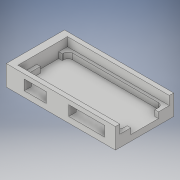
# Autodesk Inventor part: PiHolder
Saved by Autodesk Inventor 2019 (Build 230136000, 136)
## iProperties
Created: 2019-04-12
Part Number: PiHolder
Material: Generic
Document SubType Name: Modeling
Designer: Epsilon
Density: 1 g/cm^3
Appearance: Default
Author: Epsilon
Autodesk Inventor part; units mm, degrees
ref_plane "YZ Plane" through (0, 0, 0) normal (1, 0, 0) x (0, 1, 0)
ref_plane "XZ Plane" through (0, 0, 0) normal (0, 1, 0) x (-1, 0, 0)
ref_plane "XY Plane" through (0, 0, 0) normal (0, 0, 1) x (1, 0, 0)
sketch "Sketch2" plane through (0, 0, 0) normal (0, 1, 0) x (-1, 0, 0)
  line L0 (0, 0) -> (75, 0)
  line L1 (75, 0) -> (75, -40)
  line L2 (75, -40) -> (0, -40)
  line L3 (0, -40) -> (0, 0)
  dimension "d4" = 75
  dimension "d5" = 40
  constraints: 8 end point, 2 parallel, 1 horizontal, 1 perpendicular
  measures "d4" distance of L1.end L2.end
  measures "d5" distance of L0.end L1.end
extrude "Extrusion2" add sketch "Sketch2" along normal blind 14
sketch "Sketch4" plane through (0, 14, 0) normal (0, 1, 0) x (1, 0, 0)
  line L0 (0, 0) -> (0, 40) projected
  line L1 (0, 3) -> (-70, 3)
  line L2 (-70, 3) -> (-70, 37)
  line L3 (-70, 37) -> (0, 37)
  line L4 (0, 37) -> (0, 3)
  line L5 (-75, 40) -> (-75, 0) construction
  line L6 (-75, 20) -> (0, 20) construction
  dimension "d8" = 70
  dimension "d9" = 34
  constraints: 10 end point, 2 midpoint, 2 parallel, 2 perpendicular, 1 horizontal, 1 point on line, 1 other
  measures "d8" distance of L2.end L3.end
  measures "d9" distance of L1.end L2.end
extrude "Extrusion3" cut sketch "Sketch4" against normal blind 10
sketch "Sketch5" plane through (0, 4, 0) normal (0, 1, 0) x (1, 0, 0)
  line L0 (0, 3) -> (-70, 3) projected
  line L1 (-70, 37) -> (0, 37) projected
  line L2 (0, 3) -> (-70, 3)
  line L3 (-70, 3) -> (-70, 16)
  line L4 (-70, 37) -> (0, 37)
  line L5 (0, 37) -> (0, 10.475)
  line L6 (-2.5, 5) -> (-67.5, 5)
  line L7 (-67.5, 5) -> (-67.5, 16)
  line L8 (-67.5, 35) -> (-2.5, 35)
  line L9 (-2.5, 35) -> (-2.5, 29.525)
  line L10 (0, 40) -> (0, 0) construction
  line L11 (0, 20) -> (-70, 20) construction
  line L12 (-70, 3) -> (-70, 37) construction
  line L13 (-35, 3) -> (-35, 35) construction
  line L14 (0, 37) -> (0, 3) projected
  line L15 (-2.5, 10.475) -> (0, 10.475)
  line L16 (0, 29.525) -> (-2.5, 29.525)
  line L17 (-2.5, 10.475) -> (-2.5, 5)
  line L18 (0, 10.475) -> (0, 3)
  line L19 (-70, 3) -> (-70, 37) projected
  line L20 (-67.5, 31) -> (-70, 31)
  line L21 (-70, 31) -> (-70, 16) construction
  line L22 (-70, 16) -> (-67.5, 16)
  line L23 (-67.5, 16) -> (-67.5, 20) construction
  line L24 (-67.5, 31) -> (-67.5, 35)
  line L25 (-67.5, 16) -> (-67.5, 31) construction
  line L26 (-70, 16) -> (-70, 31)
  line L27 (-70, 31) -> (-70, 37)
  dimension "d12" = 65
  dimension "d13" = 30
  dimension "d17" = 19.05
  dimension "d43" = 15
  dimension "d44" = 4
  constraints: 44 end point, 17 parallel, 8 perpendicular, 4 horizontal, 4 midpoint, 3 point on line, 4 other
  measures "d12" distance of L8.start L8.end
  measures "d13" distance of L6.end L8.start
  measures "d17" distance of L16.start L5.end
  measures "d43" distance of L3.end L20.end
  measures "d44" distance between parallel lines of L8 L20
extrude "Extrusion5" add sketch "Sketch5" along normal blind 4 contours L0 L3 L22 L7 L6 L17 L15 L14 | L16 L9 L8 L24 L20 L19 L1 L5
fillet "Fillet2" radius 3 4 edges at (-2.5, 6, -5) (-67.5, 6, -5) (-67.5, 6, -35) (-2.5, 6, -35)
sketch "Sketch7" plane through (-75, 0, 0) normal (0, 0, 1) x (1, 0, 0)
  line L0 (12.4, 4) -> (27.4, 4)
  line L1 (27.4, 4) -> (27.4, 11)
  line L2 (27.4, 11) -> (12.4, 11)
  line L3 (12.4, 11) -> (12.4, 4)
  line L4 (12.4, 7.5) -> (27.4, 7.5) construction
  line L5 (19.9, 11) -> (19.9, 4) construction
  line L6 (10.5, 8) -> (10.5, 4) construction
  line L7 (10.5, 4) -> (69.5, 4) construction
  line L8 (7.5, 4) -> (7.5, 8) projected
  line L9 (42.9, 4) -> (54.9, 4)
  line L10 (54.9, 4) -> (54.9, 11) construction
  line L11 (54.9, 11) -> (42.9, 11)
  line L12 (42.9, 11) -> (42.9, 4)
  line L13 (55.5, 4) -> (67.5, 4)
  line L14 (67.5, 4) -> (67.5, 11)
  line L15 (67.5, 11) -> (55.5, 11)
  line L16 (55.5, 11) -> (55.5, 4) construction
  line L17 (48.9, 11) -> (48.9, 4) construction
  line L18 (61.5, 11) -> (61.5, 4) construction
  line L19 (54.9, 11) -> (55.5, 11) construction
  line L20 (54.9, 11) -> (55.5, 11)
  line L21 (54.9, 4) -> (55.5, 4)
  point P0 (75, 0)
  dimension "d29" = 15
  dimension "d30" = 7
  dimension "d32" = 0
  dimension "d35" = 12.4
  dimension "d36" = 12
  dimension "d37" = 7
  dimension "d38" = 12
  dimension "d39" = 7
  dimension "d40" = 41.4
  dimension "d41" = 54
  constraints: 38 end point, 8 midpoint, 6 parallel, 3 horizontal, 3 perpendicular, 2 point on line, 1 collinear
  measures "d29" distance of L2.end L1.end
  measures "d30" distance of L1.end L0.end
  measures "d32" distance between parallel lines of L7 L0
  measures "d35" distance between parallel lines of L8 L5
  measures "d36" distance of L11.end L10.end
  measures "d37" distance of L10.end L9.end
  measures "d38" distance of L15.end L14.end
  measures "d39" distance of L14.end L13.end
  measures "d40" distance between parallel lines of L8 L17
  measures "d41" distance between parallel lines of L8 L18
extrude "Extrusion7" cut sketch "Sketch7" against normal blind 6.35
equation "\"d37\" = d30"
equation "\"d38\" = d36"
equation "\"d39\" = d37"
body "Solid2"
